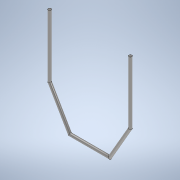
# Autodesk Inventor part: barra_palanca
Saved by Autodesk Inventor 2021 (Build 250183000, 183)
## iProperties
Created: 2022-01-26
Part Number: barra_palanca
Material: Acero, carbono
Document SubType Name: Modeling
Designer: arthu
Density: 7.85 g/cm^3
Appearance: Semipulido
Author: arthu
Autodesk Inventor part; units mm, degrees
ref_plane "YZ Plane" through (0, 0, 0) normal (1, 0, 0) x (0, 1, 0)
ref_plane "XZ Plane" through (0, 0, 0) normal (0, 1, 0) x (-1, 0, 0)
sketch "Boceto1" plane through (0, 0, 0) normal (0, 0, 1) x (1, 0, 0)
  line L0 (-332.0752, 0) -> (-331.8519, -0.5171)
  line L1 (560.0067, 1140) -> (559.9933, 1139.483)
  line L2 (332.0752, 0) -> (331.8519, -0.5171)
  line L3 (559.9933, 488.7901) -> (559.9933, 1360)
  line L4 (559.9933, 1360) -> (565.6963, 1360)
  line L5 (1679.9933, 1360) -> (1679.9933, 490)
  line L6 (1397.0917, 0) -> (842.9014, 0)
  line L7 (559.9933, 490) -> (559.9933, 1360)
  line L8 (-277.7918, 0) -> (-277.7902, -0.0027)
  line L9 (1679.9933, 1360) -> (1679.9933, 1303.9992)
  line L10 (1679.9933, 1360) -> (1679.9933, 490)
  line L11 (1679.9933, 490) -> (1397.0917, 0)
  line L12 (559.9933, 1360) -> (559.9933, 490)
  line L13 (559.9933, 490) -> (842.9014, 0)
  point P0 (0, 0)
  point P1 (0, -20)
  point P2 (277.7902, 0)
  constraints: 28 end point, 3 point on line, 2 parallel, 1 horizontal, 1 perpendicular, 1 vertical
ref_plane "Plano de trabajo6" through (1679.9933, 1360, 0) normal (0, -1, 0) x (1, 0, 0)
sketch "Boceto7" plane through (1679.9933, 1360, 0) normal (0, -1, 0) x (1, 0, 0)
  circle A0 centre (0, 0) radius 21
  circle A1 centre (0, 0) radius 19.2
  point P0 (-1679.9933, 0)
  dimension "d32" = 42
  dimension "d33" = 38.4
  constraints: 2 centre point, 1 coincident
  measures "d32" diameter of A0
  measures "d33" diameter of A1
sweep "Barrido3" add profiles "Boceto7" path "Boceto1" path curves L5 L11 L6 L13 L12
